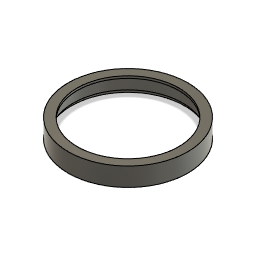
dyson_papr v3 (Autodesk Fusion 360 design; units mm, degrees)
Autodesk Fusion 360 part; units mm, degrees
sketch "Sketch1" plane through (0, 0, 0) normal (0, 1, 0) x (1, 0, 0)
  circle A0 centre (0, 0) radius 73.5
  circle A1 centre (0, 0) radius 76.5
  dimension "d1" = 147
  dimension "d2" = 3
  constraint coincident A0.centre A1.centre
  measures "d1" diameter of A0
extrude "Extrude1" add sketch "Sketch1" along normal blind 2 makes body 1
ref_plane "WorkPlane1" through (0, -17, 0) normal (0, 1, 0) x (0, 0, 1)
sketch "Sketch2" plane through (0, -17, 0) normal (0, 1, 0) x (1, 0, 0)
  circle A0 centre (0, 0) radius 76.5
  circle A1 centre (0, 0) radius 76.51
  circle A2 centre (0, 0) radius 80.5
  dimension "d10" = 0.01
  dimension "d11" = 4
extrude "Extrude2" add sketch "Sketch2" along normal blind 2 separate body contours A2 makes body 2
ref_plane "WorkPlane2" through (0, 5, 0) normal (0, 1, 0) x (1, 0, 0)
sketch "Sketch3" plane through (0, 5, 0) normal (0, 1, 0) x (1, 0, 0)
  circle A0 centre (0, 0) radius 68.5
  circle A1 centre (0, 0) radius 73.5
  circle A2 centre (0, 0) radius 80.5
  dimension "d13" = 5
  constraint coincident A0.centre A1.centre
  measures "d13" distance of A0 A1
extrude "Extrude3" add sketch "Sketch3" against normal up to surface (3 mm away) contours A1 | A2 bodies 1
sketch "Sketch4" plane through (0, 2, 0) normal (0, -1, 0) x (1, 0, 0)
  circle A0 centre (0, 0) radius 80.5
  circle A1 centre (0, 0) radius 76.5
extrude "Extrude4" add sketch "Sketch4" along normal up to surface (17 mm away) bodies 1 2
sketch "Sketch5" plane through (0, -17, 0) normal (0, -1, 0) x (1, 0, 0)
  circle A0 centre (0, 0) radius 76.51
  circle A1 centre (0, 0) radius 80.5
  circle A2 centre (0, 0) radius 76.51
extrude "Extrude5" add sketch "Sketch5" along normal blind 3 bodies 1
sketch "Sketch6" plane through (0, 0, 0) normal (0, -1, 0) x (1, 0, 0)
  circle A0 centre (0, 0) radius 73.5
  circle A1 centre (0, 0) radius 76.5
extrude "Extrude6" add sketch "Sketch6" along normal blind 15 bodies 1
